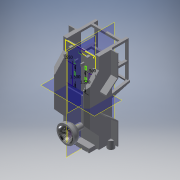
# Autodesk Inventor part: chasis
Saved by Autodesk Inventor 2019 (Build 230136000, 136)
## iProperties
Created: 2020-12-16
Part Number: chasis
Material: Generic
Document SubType Name: Modeling
Designer: saeva
Density: 1 g/cm^3
Appearance: Default
Author: saeva
Autodesk Inventor part; units mm, degrees
ref_plane "YZ Plane" through (0, 0, 0) normal (1, 0, 0) x (0, 1, 0)
ref_plane "XZ Plane" through (0, 0, 0) normal (0, 1, 0) x (-1, 0, 0)
ref_plane "XY Plane" through (0, 0, 0) normal (0, 0, 1) x (1, 0, 0)
sketch "Sketch1" plane through (0, 0, 0) normal (0, 0, 1) x (1, 0, 0)
  line L0 (-45.9342, -34.9186) -> (-29.0159, -34.9186)
  line L1 (-29.0159, -34.9186) -> (-29.0159, -54.4329)
  line L2 (-29.0159, -54.4329) -> (-45.9342, -54.4329)
  line L3 (-45.9342, -54.4329) -> (-45.9342, -34.9186)
  line L4 (-12.6528, -16.8477) -> (-23.6971, -16.8477)
  line L5 (-23.6971, -16.8477) -> (-23.6971, -4.2655)
  line L6 (-23.6971, -4.2655) -> (-12.6528, -4.2655)
  line L7 (-12.6528, -4.2655) -> (-12.6528, -16.8477)
  line L8 (-5.9423, -54.6434) -> (-9.5772, -54.6434)
  line L9 (-9.5772, -54.6434) -> (-9.5772, -34.9186)
  line L10 (-9.5772, -34.9186) -> (-5.9423, -34.9186)
  line L11 (-5.9423, -34.9186) -> (-5.9423, -54.6434)
  line L12 (0, -12.3898) -> (2.54, -12.3898)
  line L13 (2.54, -12.3898) -> (2.54, -14.9298)
  line L14 (2.54, -14.9298) -> (0, -14.9298)
  line L15 (0, -14.9298) -> (0, -12.3898)
  line L16 (-53.3526, -14.9298) -> (-55.8926, -14.9298)
  line L17 (-55.8926, -14.9298) -> (-55.8926, -12.3898)
  line L18 (-55.8926, -12.3898) -> (-53.3526, -12.3898)
  line L19 (-53.3526, -12.3898) -> (-53.3526, -14.9298)
  line L20 (-53.3526, -59.3698) -> (-55.8926, -59.3698)
  line L21 (-55.8926, -59.3698) -> (-55.8926, -56.8298)
  line L22 (-55.8926, -56.8298) -> (-53.3526, -56.8298)
  line L23 (-53.3526, -56.8298) -> (-53.3526, -59.3698)
  line L24 (0, -59.3698) -> (2.54, -59.3698)
  line L25 (2.54, -59.3698) -> (2.54, -56.8298)
  line L26 (2.54, -56.8298) -> (0, -56.8298)
  line L27 (0, -56.8298) -> (0, -59.3698)
  point P0 (0, 0)
  dimension "d11" = 2.54
  dimension "d12" = 2.54
  constraints: 56 end point, 14 parallel, 7 horizontal, 7 perpendicular, 3 point on line
  measures "d11" distance of L26.end L25.end
  measures "d12" distance of L25.end L24.end
extrude "Extrusion1" add sketch "Sketch1" along normal blind 2.54 contours L0 L1 L2 L3 | L4 L5 L6 L7 | L8 L9 L10 L11
sketch "Sketch2" plane through (0, 0, 2.54) normal (0, 0, 1) x (1, 0, 0)
  line L0 (2.8352, 2.8982) -> (-56.7679, 2.8982)
  line L1 (-56.7679, 2.8982) -> (-56.7679, -69.5579)
  line L2 (-56.7679, -69.5579) -> (2.8352, -69.5579)
  line L3 (2.8352, -69.5579) -> (2.8352, 2.8982)
  constraints: 8 end point, 2 parallel, 1 horizontal, 1 perpendicular
extrude "Extrusion2" add sketch "Sketch2" along normal blind 2.54
extrude "Extrusion3" add sketch "Sketch1" against normal blind 2.54 and the other way blind 2.54 contours L12 L13 L14 L15 | L16 L17 L18 L19 | L20 L21 L22 L23 | L27 L26 L25 L24
sketch "Sketch3" plane through (0, 0, 5.08) normal (0, 0, 1) x (1, 0, 0)
  line L0 (2.8352, 2.8982) -> (-56.7679, 2.8982) projected
  line L1 (-36.4351, 2.8982) -> (-17.5102, 2.8982)
  line L2 (2.8352, -69.5579) -> (2.8352, 2.8982) projected
  line L3 (-36.4351, -22.5439) -> (-38.7597, -22.5439)
  line L4 (-38.7597, -22.5439) -> (-38.7597, -28.5888)
  line L5 (-38.7597, -28.5888) -> (-36.4351, -28.5888)
  line L6 (-36.4351, -28.5888) -> (-36.4351, -22.5439)
  line L7 (-17.5102, -22.5439) -> (-14.6988, -22.5439)
  line L8 (-14.6988, -22.5439) -> (-14.6988, -28.5888)
  line L9 (-14.6988, -28.5888) -> (-17.5102, -28.5888)
  line L10 (-17.5102, -28.5888) -> (-17.5102, -22.5439)
  line L11 (-17.5102, -42.2194) -> (-14.6988, -42.2194)
  line L12 (-14.6988, -42.2194) -> (-14.6988, -48.7384)
  line L13 (-14.6988, -48.7384) -> (-17.5102, -48.7384)
  line L14 (-17.5102, -48.7384) -> (-17.5102, -42.2194)
  line L15 (-36.4351, -42.2194) -> (-38.7597, -42.2194)
  line L16 (-38.7597, -42.2194) -> (-38.7597, -48.7384)
  line L17 (-38.7597, -48.7384) -> (-36.4351, -48.7384)
  line L18 (-36.4351, -48.7384) -> (-36.4351, -42.2194)
  line L19 (-23.6971, -4.2655) -> (-12.6528, -4.2655) projected
  line L20 (-29.5847, -6.646) -> (-23.6971, -6.646)
  line L21 (-23.6971, -6.646) -> (-23.6971, -4.2655)
  line L22 (-23.6971, -4.2655) -> (-29.5847, -4.2655)
  line L23 (-29.5847, -4.2655) -> (-29.5847, -6.646)
  line L24 (-56.7679, 2.8982) -> (-56.7679, -69.5579) projected
  line L25 (-56.7679, -69.5579) -> (-42.7979, -69.5579)
  line L26 (-42.7979, -69.5579) -> (-42.7979, -31.4579)
  line L27 (-42.7979, -31.4579) -> (-56.7679, -31.4579)
  line L28 (-56.7679, -31.4579) -> (-56.7679, -69.5579)
  line L29 (2.8352, -69.5579) -> (-9.8648, -69.5579)
  line L30 (-9.8648, -69.5579) -> (-9.8648, -31.4579)
  line L31 (-9.8648, -31.4579) -> (2.8352, -31.4579)
  line L32 (2.8352, -31.4579) -> (2.8352, -69.5579)
  point P0 (0, 0)
  dimension "d22" = 13.97
  dimension "d24" = 38.1
  dimension "d25" = 12.7
  dimension "d26" = 38.1
  constraints: 58 end point, 14 parallel, 9 point on line, 8 horizontal, 7 perpendicular
  measures "d22" distance of L27.end L26.end
  measures "d24" distance of L25.end L26.end
  measures "d25" distance of L30.end L31.end
  measures "d26" distance of L29.end L30.end
sketch "Sketch5" plane through (2.8352, -69.5579, 2.54) normal (1, 0, 0) x (0, 0, -1)
  line L0 (-26.8295, 26.0477) -> (-2.54, 52.558)
  line L1 (-2.54, 52.558) -> (-2.54, 76.5427)
  line L2 (-2.54, 0) -> (-2.54, 72.4562) projected
  line L3 (-2.54, 76.5427) -> (22.9633, 76.5427)
  line L4 (22.9633, 76.5427) -> (22.9633, -3.7121)
  line L5 (22.9633, -3.7121) -> (-26.8295, -3.7121)
  line L6 (-26.8295, -3.7121) -> (-26.8295, 26.0477)
  line L7 (21.1811, 76.5427) -> (21.1811, 33.8528)
  line L8 (21.1811, 33.8528) -> (-0.8359, 15.4634)
  line L9 (-0.8359, 15.4634) -> (-0.8359, 12.7428)
  line L10 (0, 0) -> (0, 72.4562) projected
  line L11 (-0.8359, 12.7428) -> (22.9633, 32.6208)
  point P0 (2.54, 69.5579)
  point P1 (-2.54, 38.1)
  constraints: 20 end point, 4 perpendicular, 2 parallel, 2 point on line, 1 collinear, 1 vertical
extrude "Extrusion6" add sketch "Sketch5" along normal blind 7.62 contours L0 L1 L3 L7 L8 L9 L11 L4 L5 L6
extrude "Extrusion7" add sketch "Sketch5" along normal blind 20.32 contours L11 L10 L8 L7 L3 L4 | L11 L9 L8 L10
ref_plane "Work Plane1" through (-25.169, -69.5579, 2.54) normal (-1, 0, 0) x (0, 0, 1)
mirror "Mirror1" about plane through (-25.169, -69.5579, 2.54) normal (-1, 0, 0) of "Extrusion6", "Extrusion7"
ref_plane "Work Plane2" through (6.6452, -73.2701, -20.4233) normal (0, -1, 0) x (1, 0, 0)
mirror "Mirror2" about plane through (6.6452, -73.2701, -20.4233) normal (0, -1, 0) of "Extrusion6", "Extrusion7", "Mirror1", "Extrusion2"
sketch "Sketch7" plane through (23.1552, 6.9847, -20.4233) normal (0, 0, -1) x (-1, 0, 0)
  line L0 (12.7, -84.106) -> (83.9485, -84.106)
  line L1 (83.9485, -84.106) -> (83.9485, -156.4231)
  line L2 (83.9485, -156.4231) -> (12.7, -156.4231)
  line L3 (12.7, -156.4231) -> (12.7, -84.106)
  line L4 (83.9485, -84.106) -> (83.9485, -76.5532)
  line L5 (83.9485, -76.5532) -> (76.3285, -76.5532)
  line L6 (12.7, -76.5532) -> (12.7, -84.106)
  line L7 (83.9485, -76.5532) -> (83.9485, 0)
  line L8 (76.3285, 0) -> (76.3285, -4.0865)
  line L9 (83.9485, 0) -> (76.3285, 0)
  line L10 (76.3285, -76.5427) -> (20.32, -76.5427)
  line L11 (76.3285, 0) -> (76.3285, -76.5427)
  line L12 (20.32, -76.5427) -> (20.32, -51.1427)
  line L13 (20.32, 0) -> (20.32, -76.5427)
  line L14 (20.32, -76.5427) -> (20.32, 0)
  line L15 (12.7, 0) -> (12.7, -23.9846)
  line L16 (12.7, 0) -> (12.7, -76.5532)
  line L17 (76.3285, -76.5532) -> (20.32, -76.5532)
  line L18 (20.32, -76.5532) -> (12.7, -76.5532)
  line L19 (20.32, 0) -> (20.32, -4.0865) projected
  line L20 (12.7, 0) -> (12.7, -23.9846) projected
  line L21 (20.32, 0) -> (12.7, 0)
  constraints: 40 end point, 2 point on line, 1 parallel, 1 perpendicular
extrude "Extrusion11" add sketch "Sketch7" along normal blind 2.54 contours L16 L15 L21 L13 L12 L10 L11 L8 L9 L7 L5 L17 L18
extrude "Extrusion12" add sketch "Sketch7" along normal blind 2.54 contours L0 L1 L2 L3
chamfer "Chamfer5" distance 12.7 angle 10 2 edges at (10.4552, -113.2798, -22.9633) (-60.7933, -113.2798, -22.9633) measured on face at (-13.2943, -101.227, -22.9633)
chamfer "Chamfer6" distance 2.54 angle 45 2 edges at (10.4552, -31.2919, -22.9633) (-60.7933, -31.2919, -22.9633) measured on face at (7.9152, -44.0472, -22.9633)
sketch "Sketch8" plane through (10.4552, -69.5579, 2.54) normal (1, 0, 0) x (0, 0, -1)
  line L0 (25.5033, -7.5633) -> (25.5033, -79.8804) projected
  line L1 (22.9633, 0) -> (25.5033, 0)
  line L2 (25.5033, -7.5633) -> (22.9633, -7.5633)
  line L3 (22.9633, -7.5633) -> (22.9633, 0)
  line L4 (25.5033, 0) -> (59.2283, 5.3826)
  line L5 (59.2283, 5.3826) -> (59.2283, 1.8542)
  line L6 (59.2283, 1.8542) -> (25.5033, -7.5633)
  point P0 (2.54, 69.5579)
  constraints: 12 end point, 1 horizontal, 1 parallel, 1 vertical
extrude "Extrusion13" add sketch "Sketch8" against normal blind 71.247
chamfer "Chamfer7" distance 6.35 angle 45 2 edges at (10.4552, -73.2701, 29.3695) (-60.7933, -73.2701, 29.3695)
sketch "Sketch9" plane through (-53.1733, -149.4384, -20.4233) normal (0, -1, 0) x (1, 0, 0)
  line L0 (56.0085, 0) -> (56.0085, -2.54) projected
  line L1 (0, 25.5033) -> (0, 49.7928) projected
  line L2 (56.0085, -1.27) -> (0, -1.27)
  line L3 (0, -1.27) -> (0, 37.6481)
  line L4 (0, 37.6481) -> (56.0085, 37.6481)
  line L5 (56.0085, 37.6481) -> (56.0085, -1.27)
  point P0 (53.1733, 20.4233)
  constraints: 8 end point, 2 midpoint, 2 parallel, 1 horizontal, 1 perpendicular
extrude "Extrusion14" add sketch "Sketch9" along normal blind 7.747
sketch "Sketch10" plane through (23.1552, 6.9847, -22.9633) normal (0, 0, -1) x (-1, 0, 0)
  line L0 (81.4085, 0) -> (81.4085, -4.0865)
  line L1 (20.32, -4.1142) -> (15.3131, -4.1142)
  line L2 (15.3131, -4.1142) -> (15.3131, 0)
  line L3 (76.3285, 0) -> (76.3285, -4.0865)
  line L4 (76.3285, 0) -> (76.3285, -4.0865)
  line L5 (20.32, -4.1142) -> (20.32, 0)
  line L6 (15.3131, 0) -> (20.32, 0)
  line L7 (76.3285, 0) -> (81.4085, 0)
  line L8 (76.3285, -4.0865) -> (81.4085, -4.0865)
  line L9 (15.3131, -42.2142) -> (15.3131, -38.1)
  line L10 (15.3131, -38.1) -> (20.32, -38.1)
  line L11 (20.32, -42.2142) -> (15.3131, -42.2142)
  line L12 (20.32, -42.2142) -> (20.32, -38.1)
  line L13 (76.3285, -38.1) -> (76.3285, -42.1865)
  line L14 (76.3285, -38.1) -> (81.4085, -38.1)
  line L15 (76.3285, -42.1865) -> (81.4085, -42.1865)
  line L16 (81.4085, -38.1) -> (81.4085, -42.1865)
  point P0 (23.1552, -6.9847)
  dimension "d70" = 38.1
  constraints: 34 end point, 3 parallel, 2 collinear, 2 horizontal, 2 perpendicular, 1 vertical, 15 other
  measures "d70" distance of L1.end L9.start
extrude "Extrusion15" add sketch "Sketch10" along normal blind 33.7312
sketch "Sketch12" plane through (2.8352, -69.5579, 2.54) normal (-1, 0, 0) x (0, 0, 1)
  line L0 (-25.5033, 34.3285) -> (-59.2345, 34.3285) projected
  line L1 (-25.5033, 38.4427) -> (-59.2345, 38.4427) projected
  line L2 (-49.7505, 34.3285) -> (-45.6357, 34.3285)
  line L3 (-45.6357, 34.3285) -> (-45.6357, 38.4427)
  line L4 (-45.6357, 38.4427) -> (-49.7505, 38.4427)
  line L5 (-49.7505, 38.4427) -> (-49.7505, 34.3285)
  line L6 (-45.6357, 76.5427) -> (-49.7505, 76.5427)
  line L7 (-45.6357, 72.4285) -> (-45.6357, 76.5427)
  line L8 (-49.7505, 72.4285) -> (-45.6357, 72.4285)
  line L9 (-49.7505, 76.5427) -> (-49.7505, 72.4285)
  point P0 (-2.54, 69.5579)
  dimension "d80" = 4.1148
  dimension "d83" = 38.1
  constraints: 16 end point, 2 parallel, 2 point on line, 1 collinear, 1 horizontal, 1 perpendicular, 1 vertical, 7 other
  measures "d80" distance of L4.end L3.end
  measures "d83" distance of L3.end L6.start
extrude "Extrusion17" add sketch "Sketch12" along normal blind 56.007
sketch "Sketch13" plane through (-58.2533, 2.8982, -22.9633) normal (0, -1, 0) x (1, 0, 0)
  line L0 (66.0954, -33.7312) -> (61.0885, -33.7312) projected
  line L1 (61.0885, -24.2472) -> (61.0885, -33.7312) projected
  line L2 (66.0954, -33.7312) -> (61.0885, -33.7312)
  line L3 (61.0885, -33.7312) -> (61.0885, -31.2835)
  line L4 (61.0885, -31.2835) -> (66.0954, -31.2835)
  line L5 (66.0954, -31.2835) -> (66.0954, -33.7312)
  line L6 (5.08, 0) -> (5.08, -33.7312) projected
  line L7 (5.08, -33.7312) -> (0.0769, -33.7312)
  line L8 (0.0769, -33.7312) -> (0.0769, -31.2835)
  line L9 (0.0769, -31.2835) -> (5.08, -31.2835)
  line L10 (5.08, -31.2835) -> (5.08, -33.7312)
  point P0 (58.2533, 22.9633)
  dimension "d90" = 2.4477
  constraints: 16 end point, 4 parallel, 2 horizontal, 2 perpendicular, 1 point on line
  measures "d90" distance of L4.end L0.start
extrude "Extrusion18" add sketch "Sketch13" along normal blind 67.1195
sketch "Sketch14" plane through (-58.2533, -64.2213, -22.9633) normal (0, -1, 0) x (1, 0, 0)
  line L0 (68.7085, -33.7249) -> (-2.5385, -33.7249) projected
  line L1 (21.8388, -33.7249) -> (43.3735, -33.7249)
  line L2 (43.3735, -33.7249) -> (43.3735, -30.7008)
  line L3 (43.3735, -30.7008) -> (21.8388, -30.7008)
  line L4 (21.8388, -30.7008) -> (21.8388, -33.7249)
  point P0 (58.2533, 22.9633)
  constraints: 8 end point, 2 parallel, 1 horizontal, 1 perpendicular, 1 point on line
extrude "Extrusion19" add sketch "Sketch14" along normal blind 1.016 and the other way blind 0.508
chamfer "Chamfer8" distance 3.175 angle 45 1 edges at (-25.169, -157.1854, -21.6933)
sketch "Sketch15" plane through (-53.1733, -157.1854, -20.4233) normal (0, -1, 0) x (1, 0, 0)
  line L0 (0, 37.6481) -> (56.0085, 37.6481) projected
  line L1 (56.0085, 1.905) -> (0, 1.905) projected
  line L2 (53.1733, 37.6481) -> (50.7097, 37.6481)
  line L3 (50.7097, 37.6481) -> (50.7097, 1.905)
  line L4 (50.7097, 1.905) -> (53.1733, 1.905)
  line L5 (53.1733, 1.905) -> (53.1733, 37.6481)
  line L6 (39.2797, 37.6481) -> (39.2797, 1.905)
  line L7 (39.2797, 1.905) -> (41.7433, 1.905)
  line L8 (41.7433, 1.905) -> (41.7433, 37.6481)
  line L9 (41.7433, 37.6481) -> (39.2797, 37.6481)
  line L10 (27.8497, 37.6481) -> (27.8497, 1.905)
  line L11 (27.8497, 1.905) -> (30.3133, 1.905)
  line L12 (30.3133, 1.905) -> (30.3133, 37.6481)
  line L13 (30.3133, 37.6481) -> (27.8497, 37.6481)
  line L14 (16.4197, 37.6481) -> (16.4197, 1.905)
  line L15 (16.4197, 1.905) -> (18.8833, 1.905)
  line L16 (18.8833, 1.905) -> (18.8833, 37.6481)
  line L17 (18.8833, 37.6481) -> (16.4197, 37.6481)
  line L18 (4.9897, 37.6481) -> (4.9897, 1.905)
  line L19 (4.9897, 1.905) -> (7.4533, 1.905)
  line L20 (7.4533, 1.905) -> (7.4533, 37.6481)
  line L21 (7.4533, 37.6481) -> (4.9897, 37.6481)
  point P0 (53.1733, 20.4233)
  dimension "d102" = 11.43
  constraints: 40 end point, 2 horizontal, 2 parallel, 2 point on line, 1 perpendicular, 32 other
  measures "d102" distance of L2.end L6.start
extrude "Extrusion20" cut sketch "Sketch15" against normal blind 1.016 contours L0 L20 L1 L18 | L0 L16 L1 L14 | L0 L12 L1 L10 | L0 L8 L1 L6 | L0 L5 L1 L3
sketch "Sketch16" plane through (-60.7918, -67.7037, -56.6883) normal (0, -0.9631528, -0.2689549) x (1, 0, 0)
  line L0 (66.167, 32.2372) -> (5.6899, 32.2372)
  line L1 (5.6899, 32.2372) -> (5.6899, 2.276)
  line L2 (5.6899, 2.276) -> (66.167, 2.276)
  line L3 (66.167, 2.276) -> (66.167, 32.2372)
  point P0 (60.7918, 36.3902)
  constraints: 8 end point, 2 parallel, 1 horizontal, 1 perpendicular
extrude "Extrusion21" cut sketch "Sketch16" against normal blind 7.62
sketch "Sketch17" plane through (-73.4933, -153.5249, -18.6411) normal (0, -1, 0) x (1, 0, 0)
  line L0 (12.7, 0) -> (0, 0) projected
  circle A0 centre (12.7, 0) radius 6.35
  line L1 (83.9485, 0) -> (83.9485, 23.7211) projected
  circle A1 centre (83.9485, 0) radius 6.35
  point P0 (73.4933, 18.6411)
  dimension "d111" = 12.7
  dimension "d112" = 12.7
  constraints: 2 centre point
  measures "d111" diameter of A0
  measures "d112" diameter of A1
extrude "Extrusion22" add sketch "Sketch17" along normal mid plane 15.24
sketch "Sketch18" plane through (-60.7933, -161.1449, -18.6411) normal (0, -1, 0) x (1, 0, 0)
  line L0 (71.2485, 0) -> (83.9485, 0) projected
  line L1 (71.2485, -4.3223) -> (71.2485, -2.0829) projected
  circle A0 centre (71.2485, 0) radius 4.3223
  line L2 (0.0015, -4.3223) -> (0.0015, -2.0832) projected
  circle A1 centre (0, 0) radius 4.3223
  point P0 (60.7933, 18.6411)
  constraints: 1 vertical alignment, 5 other
extrude "Extrusion23" cut sketch "Sketch18" against normal blind 5.08
sketch "Sketch20" plane through (0, 0, 5.08) normal (0, 0, 1) x (1, 0, 0)
  line L0 (2.8352, -31.1153) -> (2.8352, 2.8706) projected
  line L1 (2.8352, -17.0169) -> (0.8745, -17.0169)
  line L2 (0.8745, -17.0169) -> (0.8745, -21.8486)
  line L3 (0.8745, -21.8486) -> (2.8352, -21.8486)
  line L4 (2.8352, -21.8486) -> (2.8352, -17.0169)
  line L5 (-18.0913, -17.0169) -> (-20.5676, -17.0169)
  line L6 (-20.5676, -17.0169) -> (-20.5676, -21.8486)
  line L7 (-20.5676, -21.8486) -> (-18.0913, -21.8486)
  line L8 (-18.0913, -21.8486) -> (-18.0913, -17.0169)
  line L9 (-6.0828, 0) -> (-10.8678, 0)
  line L10 (-10.8678, 0) -> (-10.8678, -2.1529)
  line L11 (-10.8678, -2.1529) -> (-6.0828, -2.1529)
  line L12 (-6.0828, -2.1529) -> (-6.0828, 0)
  line L13 (-53.1733, 2.8982) -> (-53.1733, -31.1153) projected
  point P0 (0, 0)
  constraints: 24 end point, 6 parallel, 3 horizontal, 3 perpendicular, 1 point on line
ref_plane "Work Plane3" through (-25.169, -17.0169, 17.78) normal (-1, 0, 0) x (0, 0, 1)
extrude "Extrusion25" add sketch "Sketch20" along normal blind 6.35
mirror "Mirror3" about plane through (-25.169, -17.0169, 17.78) normal (-1, 0, 0) of "Extrusion25"
sketch "Sketch24" plane through (-53.1733, -76.9822, 5.08) normal (0, 0, 1) x (1, 0, 0)
  line L0 (56.0085, -52.558) -> (63.6285, -52.558) projected
  line L1 (0, -52.558) -> (0, -26.0477) projected
  line L2 (56.0085, -52.558) -> (0, -52.558)
  circle A0 centre (28.0043, -52.558) radius 5.6966
  point P0 (53.1733, 76.9822)
  constraints: 2 end point, 1 centre point, 1 horizontal, 1 midpoint
extrude "Extrusion28" add sketch "Sketch24" along normal blind 15.875
ref_plane "Work Plane4" through (-25.169, -135.2368, 20.955) normal (1, 0, 0) x (0, 0, -1)
sketch "Sketch26" plane through (-25.169, -135.2368, 20.955) normal (1, 0, 0) x (0, 0, -1)
  line L0 (0, 11.3932) -> (0, 0) projected
  arc A0 (0, 5.6966) -> (-14.8503, 20.5469) centre (-14.8503, 5.6966) ccw
  arc A1 (4.1936, 5.6966) -> (-8.6375, 23.6986) centre (-14.8503, 5.6966) ccw
  line L1 (0, 5.6966) -> (4.1936, 5.6966)
  line L2 (-14.8503, 20.5469) -> (-14.8503, 23.6986)
  line L3 (-14.8503, 23.6986) -> (-8.6375, 23.6986)
  point P0 (20.955, 135.2368)
  constraints: 6 end point, 4 point on circle, 2 centre point, 2 coincident, 1 horizontal, 1 midpoint, 1 vertical
revolve "Revolution1" add sketch "Sketch26" angle 360 about axis through (-25.169, -129.5402, 20.955) along (0, 0, -1)
body "Solid1"
